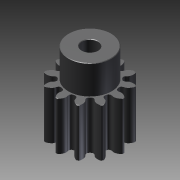
# Autodesk Inventor part: GEAHBB3.0-12-30-B-10_b
Saved by Autodesk Inventor 2011 SP1 (Build 150282100, 282)
## iProperties
Created: 2016-11-09
Part Number: GEAHBB3.0-12-30-B-10_b
Catalog Web Link: www.cadenas.de
Description: GEAHB, GEAHBB, GEAHS, GEAB, GEABB, GEABG, GEAKB, GEAKBB, GEAKBG_3.0_body-Spur Gears - Pressure Angle 20 degree Module 3.0
Vendor: MISUMI
Document SubType Name: Modeling
Designer: psAdmin
Manufacturer: MISUMI
Mass: 35.4987 g
Surface Area: 113.85 cm^2
Volume: 35.4987 cm^3
Density: 1 g/cm^3
Category: PARTsolutions
Company: MISUMI
Title: GEAHBB3.0-12-30-B-10
Author: Cadenas PARTsolutions
Comments: Spur Gears - Pressure Angle 20 degree Module 3.0
PSOL_IDENT_0: {$CADENAS_DATA\23d-libs\misumi\metric\54_spur_gears\geahb30\geahb30.prj},413 {VTYP=3D},{NB=GEAHBB3.0
PSOL_IDENT_1: -12-30-B-10_b},{LINA=GEAHBB3.0-12-30-B-10},{NN=GEAHB, GEAHBB, GEAHS, GEAB, GEABB, GEABG, GEAKB, GEAK
PSOL_IDENT_2: BB, GEAKBG_3.0_body},{DATE=13.09.2016 11:21:23},{GEOMDATE=13.09.2016 06:20:28},{VERSION=},{LINEID=10
PSOL_IDENT_3: },{LINESUBID=-1},{WBVAR=SHS,MAT,ST,NT,TS,PS,ALT1,ALT2,TPC,ALT11,ALT10,BS,ALT4,Z,J,ALT5,Q,R,S,T,ALT9,
PSOL_IDENT_4: SRG,ALT6,LFC,LTC,MALT6,ALT7,KFC,KTC,K,ALT3,DIRALT3,QFC,QTC,MALT3,ALT8,DIRALT8,ZFC,ZTC,U}  {NB=GEAHBB
PSOL_IDENT_5: 3.0-12-30-B-10_b},{LINA=GEAHBB3.0-12-30-B-10},{KT=DUMMY},{PN=GEAHBB3.0-12-30-B-10},{TYPE=GEAHBB},{SH
PSOL_IDENT_6: S=RH},{SHSALG= 'RH','Round Hole','KGH','Key Groove Hole','KGHT','Key Groove Hole+Tap' },{SHALG=1},{S
PSOL_IDENT_7: HSPN=RH},{GEAK=2},{MAT=S45C},{MATALG= 'S45C', 'S45C Equivalent', 'SUS304', 'SUS304' },{ST=BO},{STALG=
PSOL_IDENT_8: '','-','BO','Black Oxide','ENP','Electroless Nickel Plating'},{AC=-},{MOD=3.0},{NT=12},{NTA=[12,14,
PSOL_IDENT_9: 15,16,17,18,19,20,21,22,23,24,25,26,27,28,29,30,32,34,35,36,38,40,42,44,45,46,48,50,52,54,55,56,58,6
PSOL_IDENT_10: 0,62,64,65,68,70]},{B=30},{TS=B},{TSALG='A','A','B','B'},{TSPN=-B},{PS=10},{PSA='8','8','9','9','10'
PSOL_IDENT_11: ,'10','11','11','12','12','13','13','14','14','15','15','16','16','17','17'},{PSA1='8','8','9','9','
PSOL_IDENT_12: 10','10','11','11','12','12','13','13','14','14','15','15','16','16','17','17'},{PSA2='8N','8N','10N'
PSOL_IDENT_13: ,'10N','10K','10K','11N','11N','12N','12N'},{P=10.000},{P2=10},{DD=36.0},{D=42.0},{G=28.5},{H=27},{L=
PSOL_IDENT_14: 48},{LL1=18},{LL2=9},{M=-},{M2=6},{BB=0},{TT=0},{ALT1=},{ALT1ALG= '','N/A' },{ALT1PN=},{ALT2=},{ALT2
PSOL_IDENT_15: ALG= '','N/A' },{TPC=N/A},{TPCALG= 'N/A' },{ALT2PN=},{KC=0},{ALT11=},{ALT11ALG= '','N/A' },{ALT11PN=
PSOL_IDENT_16: },{DEG=0},{ALT10=},{ALT10ALG= '','w/o BS (Boss Cut)','BS','with BS (Boss Cut)' },{BS=0.0},{BSALG=0},
PSOL_IDENT_17: {BSMIN=3},{BSMAX=18},{ALT10PN=},{LL13D=18.000},{LL23D=39.000},{LBS=48.000},{ALT4=},{ALT4ALG='','w/o
PSOL_IDENT_18: Stepped Hole','DHL','with DHL (Stepped Hole)','DHR','with DHR (Stepped Hole)'},{ALT4PN=},{ALT41=1},{
PSOL_IDENT_19: ALT42=1},{Z=0},{ZALG=0},{ZMINL=12},{ZMAXL=24},{ZMINR=12},{ZMAXR=23},{ZPN=},{J=0.0},{JALG=0},{JMIN=2}
PSOL_IDENT_20: ,{JMAX=0},{JPN=},{ALT5=},{ALT5ALG= '','w/o WDH (Both Ends Stepped Hole)','WDH','with WDH (Both Ends
PSOL_IDENT_21: Stepped Hole)' },{ALT5PN=},{Q=0},{QALG=0},{QMIN=12},{QMAX=23},{QPN=},{R=0},{RALG=0},{RMIN=12},{RMAX=
PSOL_IDENT_22: 23},{RPN=},{S=0},{SALG=0},{SMIN=3},{SMAX=42},{SPN=},{T=0},{TALG=0},{TMIN=3},{TMAX=0},{TPN=},{ALT9=},
PSOL_IDENT_23: {ALT9ALG= '','Not applicable' },{SRG=0.0},{SRGALG=0},{SRGMIN=3.500},{SRGMINALG=3.500},{SRGMAX=0.000}
PSOL_IDENT_24: ,{SRGMAXALG=0.000},{DD2=0.0},{MM=0.00},{NN=0.00},{DD2ALG=0.000},{MMALG=0.000},{NNALG=0.000},{ALT9PN=
PSOL_IDENT_25: },{ALT6=},{ALT6ALG= '','Not applicable' },{LFC=0},{LFCALG=0},{LTC=0},{LTCALG=0},{LPCDMIN=18},{LPCDMA
PSOL_IDENT_26: X=21},{MALT6=N/A},{MALT6ALG= 'N/A' },{C=0.0},{ALT6PN=},{ALT7=},{ALT7ALG= '','w/o Side Through Hole','
PSOL_IDENT_27: KFC','with KFC (Side Through Hole)','KTC','with KTC (Side Through Hole)' },{ALT7PN=},{KPCDMIN1=17},{
PSOL_IDENT_28: KPCDMAX1=20},{KPCDMIN2=34},{KPCDMAX2=21},{KFC=0},{KFCALG=[0]},{KTC=0},{KTCALG=[0]},{K=0.0},{KALG=[0]
PSOL_IDENT_29: },{KALT7L=30},{KPCD=0},{TIF=2},{SCREW=0.000},{SCREWL=0},{PLANE=13.5},{PLANE1=13.5},{ALT3=},{ALT3ALG=
PSOL_IDENT_30: '','w/o Side Tapped Hole','QFC','with QFC (Side Tapped Hole)','QTC','with QTC (Side Tapped Hole)' }
PSOL_IDENT_31: ,{ALT3PN=},{DIRALT3=},{DIRALT3ALG= '','N/A' },{QFC=0},{QFCALG=[0]},{QTC=0},{QTCALG=[0]},{QPCDMIN1=17
PSOL_IDENT_32: },{QPCDMAX1=20},{QPCDMIN2=34},{QPCDMAX2=21},{CIFMALT3=3},{QPCD=0},{MALT3=N/A},{MALT3ALG= 'N/A' },{MA
PSOL_IDENT_33: LT3L=0},{PITCH=0},{MS1=3},{ALT8=},{ALT8ALG= '','Not applicable' },{ALT8PN=},{DIRALT8=},{DIRALT8ALG= ''
PSOL_IDENT_34: ,'N/A' },{ZFC=0},{ZFCALG=[0]},{ZTC=0},{ZTCALG=[0]},{ZPCDMIN1=20},{ZPCDMIN2=38},{ZPCDMAX1=16},{ZPCDMA
PSOL_IDENT_35: X2=18},{ZPCD=0},{U=0},{UMAX=0},{UALG=[0]},{UMAX1=0},{UMAX2=6},{UMIN=3},{U1=0.0},{U2=0.0},{F=0.0},{PC
PSOL_IDENT_36: D=0},{PZQRDD2=10},{SHN=0},{SHDEG1=0},{SHDEG2=0},{ALT3LBS=47.5},{ML=0},{MOD3D=3},{D1=7.5},{D2=15},{D3=
PSOL_IDENT_37: 20},{D4=0.3},{D5=6},{D6=3.692308},{D7=2.55},{D8=1.5},{D9=2.406515},{S1=15},{S2=0.5}
NN: 0.00
NT: 12
NB: GEAHBB3.0-12-30-B-10_b
NBSYN: $PN._b
LINA: GEAHBB3.0-12-30-B-10
PN: GEAHBB3.0-12-30-B-10
SHS: Round Hole
MAT: S45C Equivalent
ST: Black Oxide
MOD: 3.0
B: 30
TS: B
PS: 10
DD: 36.0
D: 42.0
G: 28.5
H: 27
L: 48
LL1: 18
LL2: 9
M: -
ALT1: N/A
ALT2: N/A
TPC: N/A
ALT11: N/A
ALT10: w/o BS (Boss Cut)
BS: 0.0
ALT4: w/o Stepped Hole
Z: 0
J: 0.0
ALT5: w/o WDH (Both Ends Stepped Hole)
Q: 0
R: 0
S: 0
T: 0
ALT9: Not applicable
SRG: 0.0
DD2: 0.0
MM: 0.00
ALT6: Not applicable
LFC: 0
LTC: 0
MALT6: N/A
C: 0.0
ALT7: w/o Side Through Hole
KFC: 0
KTC: 0
K: 0.0
ALT3: w/o Side Tapped Hole
DIRALT3: N/A
QFC: 0
QTC: 0
MALT3: N/A
ALT8: Not applicable
DIRALT8: N/A
ZFC: 0
ZTC: 0
U: 0
U1: 0.0
U2: 0.0
F: 0.0
SUPPLIER: MISUMI
ARTICLENO: GEAHBB3.0-12-30-B-10_b
BOMINFO: GEAHBB3.0-12-30-B-10
CREATOR: CADENAS GmbH
Autodesk Inventor part; units mm, degrees
sketch "Sketch_2" plane through (0, 0, 0) normal (1, 0, 0) x (0, 1, 0)
  line L0 (0, -500) -> (0, 500)
  line L1 (0, 48) -> (13.2, 48)
  line L2 (13.2, 48) -> (13.5, 47.7)
  line L3 (13.5, 47.7) -> (13.5, 30)
  line L4 (13.5, 30) -> (20.5, 30)
  line L5 (20.5, 30) -> (26, 28.5263)
  line L6 (26, 28.5263) -> (26, 1.4737)
  line L7 (26, 1.4737) -> (20.5, 0)
  line L8 (20.5, 0) -> (0, 0)
  line L9 (0, 0) -> (0, 48)
  constraints: 20 end point
revolve "Revolution1" add sketch "Sketch_2" angle 360 about axis through (0, 0, -500) along (0, 0, -1)
sketch "Sketch_3" plane through (0, 0, 0) normal (0, 0, 1) x (1, 0, 0)
  circle A0 centre (0, 0) radius 84
  arc A1 (-20.9961, 0.4062) -> (-20.9961, -0.4062) centre (0, 0) ccw
  arc A2 (-20.9961, -0.4062) -> (-20.9145, -0.6061) centre (-20.6961, -0.4004) ccw
  arc A3 (-20.9145, -0.6061) -> (-17.846, -2.3495) centre (-16.5474, 3.5083) ccw
  arc A4 (-17.846, -2.3495) -> (-16.611, -2.2981) centre (-17.3251, 0) ccw
  arc A5 (-15.1899, -2.1473) -> (-16.611, -2.2981) centre (-15.5182, -5.825) ccw
  arc A6 (-13.8639, -3.2946) -> (-15.1899, -2.1473) centre (-15.3233, -3.6414) ccw
  arc A7 (-13.8639, -3.2946) -> (-13.6538, -4.0788) centre (0, 0) ccw
  arc A8 (-14.2285, -5.7353) -> (-13.6538, -4.0788) centre (-15.091, -4.5081) ccw
  arc A9 (-15.5346, -6.3153) -> (-14.2285, -5.7353) centre (-16.3516, -2.7145) ccw
  arc A10 (-15.5346, -6.3153) -> (-16.6298, -6.8883) centre (-15.004, -8.6626) ccw
  arc A11 (-16.6298, -6.8883) -> (-18.4155, -9.9323) centre (-12.5763, -11.312) ccw
  arc A12 (-18.4155, -9.9323) -> (-18.3862, -10.1463) centre (-18.1236, -10.0013) ccw
  arc A13 (-18.3862, -10.1463) -> (-17.98, -10.8498) centre (0, 0) ccw
  arc A14 (-17.98, -10.8498) -> (-17.8094, -10.9821) centre (-17.7232, -10.6948) ccw
  arc A15 (-17.8094, -10.9821) -> (-14.2804, -10.9577) centre (-16.0846, -5.2354) ccw
  arc A16 (-14.2804, -10.9577) -> (-13.2365, -10.2957) centre (-15.004, -8.6626) ccw
  arc A17 (-12.0812, -9.4546) -> (-13.2365, -10.2957) centre (-10.5266, -12.8037) ccw
  arc A18 (-10.3592, -9.7851) -> (-12.0812, -9.4546) centre (-11.4497, -10.8152) ccw
  arc A19 (-10.3592, -9.7851) -> (-9.7851, -10.3592) centre (0, 0) ccw
  arc A20 (-9.4546, -12.0812) -> (-9.7851, -10.3592) centre (-10.8152, -11.4497) ccw
  arc A21 (-10.2957, -13.2365) -> (-9.4546, -12.0812) centre (-12.8037, -10.5266) ccw
  arc A22 (-10.2957, -13.2365) -> (-10.9577, -14.2804) centre (-8.6626, -15.004) ccw
  arc A23 (-10.9577, -14.2804) -> (-10.9821, -17.8094) centre (-5.2354, -16.0846) ccw
  arc A24 (-10.9821, -17.8094) -> (-10.8498, -17.98) centre (-10.6948, -17.7232) ccw
  arc A25 (-10.8498, -17.98) -> (-10.1463, -18.3862) centre (0, 0) ccw
  arc A26 (-10.1463, -18.3862) -> (-9.9323, -18.4155) centre (-10.0013, -18.1236) ccw
  arc A27 (-9.9323, -18.4155) -> (-6.8883, -16.6298) centre (-11.312, -12.5763) ccw
  arc A28 (-6.8883, -16.6298) -> (-6.3153, -15.5346) centre (-8.6626, -15.004) ccw
  arc A29 (-5.7353, -14.2285) -> (-6.3153, -15.5346) centre (-2.7145, -16.3516) ccw
  arc A30 (-4.0788, -13.6538) -> (-5.7353, -14.2285) centre (-4.5081, -15.091) ccw
  arc A31 (-4.0788, -13.6538) -> (-3.2946, -13.8639) centre (0, 0) ccw
  arc A32 (-2.1473, -15.1899) -> (-3.2946, -13.8639) centre (-3.6414, -15.3233) ccw
  arc A33 (-2.2981, -16.611) -> (-2.1473, -15.1899) centre (-5.825, -15.5182) ccw
  arc A34 (-2.2981, -16.611) -> (-2.3495, -17.846) centre (0, -17.3251) ccw
  arc A35 (-2.3495, -17.846) -> (-0.6061, -20.9145) centre (3.5083, -16.5474) ccw
  arc A36 (-0.6061, -20.9145) -> (-0.4062, -20.9961) centre (-0.4004, -20.6961) ccw
  arc A37 (-0.4062, -20.9961) -> (0.4062, -20.9961) centre (0, 0) ccw
  arc A38 (0.4062, -20.9961) -> (0.6061, -20.9145) centre (0.4004, -20.6961) ccw
  arc A39 (0.6061, -20.9145) -> (2.3495, -17.846) centre (-3.5083, -16.5474) ccw
  arc A40 (2.3495, -17.846) -> (2.2981, -16.611) centre (0, -17.3251) ccw
  arc A41 (2.1473, -15.1899) -> (2.2981, -16.611) centre (5.825, -15.5182) ccw
  arc A42 (3.2946, -13.8639) -> (2.1473, -15.1899) centre (3.6414, -15.3233) ccw
  arc A43 (3.2946, -13.8639) -> (4.0788, -13.6538) centre (0, 0) ccw
  arc A44 (5.7353, -14.2285) -> (4.0788, -13.6538) centre (4.5081, -15.091) ccw
  arc A45 (6.3153, -15.5346) -> (5.7353, -14.2285) centre (2.7145, -16.3516) ccw
  arc A46 (6.3153, -15.5346) -> (6.8883, -16.6298) centre (8.6626, -15.004) ccw
  arc A47 (6.8883, -16.6298) -> (9.9323, -18.4155) centre (11.312, -12.5763) ccw
  arc A48 (9.9323, -18.4155) -> (10.1463, -18.3862) centre (10.0013, -18.1236) ccw
  arc A49 (10.1463, -18.3862) -> (10.8498, -17.98) centre (0, 0) ccw
  arc A50 (10.8498, -17.98) -> (10.9821, -17.8094) centre (10.6948, -17.7232) ccw
  arc A51 (10.9821, -17.8094) -> (10.9577, -14.2804) centre (5.2354, -16.0846) ccw
  arc A52 (10.9577, -14.2804) -> (10.2957, -13.2365) centre (8.6626, -15.004) ccw
  arc A53 (9.4546, -12.0812) -> (10.2957, -13.2365) centre (12.8037, -10.5266) ccw
  arc A54 (9.7851, -10.3592) -> (9.4546, -12.0812) centre (10.8152, -11.4497) ccw
  arc A55 (9.7851, -10.3592) -> (10.3592, -9.7851) centre (0, 0) ccw
  arc A56 (12.0812, -9.4546) -> (10.3592, -9.7851) centre (11.4497, -10.8152) ccw
  arc A57 (13.2365, -10.2957) -> (12.0812, -9.4546) centre (10.5266, -12.8037) ccw
  arc A58 (13.2365, -10.2957) -> (14.2804, -10.9577) centre (15.004, -8.6626) ccw
  arc A59 (14.2804, -10.9577) -> (17.8094, -10.9821) centre (16.0846, -5.2354) ccw
  arc A60 (17.8094, -10.9821) -> (17.98, -10.8498) centre (17.7232, -10.6948) ccw
  arc A61 (17.98, -10.8498) -> (18.3862, -10.1463) centre (0, 0) ccw
  arc A62 (18.3862, -10.1463) -> (18.4155, -9.9323) centre (18.1236, -10.0013) ccw
  arc A63 (18.4155, -9.9323) -> (16.6298, -6.8883) centre (12.5763, -11.312) ccw
  arc A64 (16.6298, -6.8883) -> (15.5346, -6.3153) centre (15.004, -8.6626) ccw
  arc A65 (14.2285, -5.7353) -> (15.5346, -6.3153) centre (16.3516, -2.7145) ccw
  arc A66 (13.6538, -4.0788) -> (14.2285, -5.7353) centre (15.091, -4.5081) ccw
  arc A67 (13.6538, -4.0788) -> (13.8639, -3.2946) centre (0, 0) ccw
  arc A68 (15.1899, -2.1473) -> (13.8639, -3.2946) centre (15.3233, -3.6414) ccw
  arc A69 (16.611, -2.2981) -> (15.1899, -2.1473) centre (15.5182, -5.825) ccw
  arc A70 (16.611, -2.2981) -> (17.846, -2.3495) centre (17.3251, 0) ccw
  arc A71 (17.846, -2.3495) -> (20.9145, -0.6061) centre (16.5474, 3.5083) ccw
  arc A72 (20.9145, -0.6061) -> (20.9961, -0.4062) centre (20.6961, -0.4004) ccw
  arc A73 (20.9961, -0.4062) -> (20.9961, 0.4062) centre (0, 0) ccw
  arc A74 (20.9961, 0.4062) -> (20.9145, 0.6061) centre (20.6961, 0.4004) ccw
  arc A75 (20.9145, 0.6061) -> (17.846, 2.3495) centre (16.5474, -3.5083) ccw
  arc A76 (17.846, 2.3495) -> (16.611, 2.2981) centre (17.3251, 0) ccw
  arc A77 (15.1899, 2.1473) -> (16.611, 2.2981) centre (15.5182, 5.825) ccw
  arc A78 (13.8639, 3.2946) -> (15.1899, 2.1473) centre (15.3233, 3.6414) ccw
  arc A79 (13.8639, 3.2946) -> (13.6538, 4.0788) centre (0, 0) ccw
  arc A80 (14.2285, 5.7353) -> (13.6538, 4.0788) centre (15.091, 4.5081) ccw
  arc A81 (15.5346, 6.3153) -> (14.2285, 5.7353) centre (16.3516, 2.7145) ccw
  arc A82 (15.5346, 6.3153) -> (16.6298, 6.8883) centre (15.004, 8.6626) ccw
  arc A83 (16.6298, 6.8883) -> (18.4155, 9.9323) centre (12.5763, 11.312) ccw
  arc A84 (18.4155, 9.9323) -> (18.3862, 10.1463) centre (18.1236, 10.0013) ccw
  arc A85 (18.3862, 10.1463) -> (17.98, 10.8498) centre (0, 0) ccw
  arc A86 (17.98, 10.8498) -> (17.8094, 10.9821) centre (17.7232, 10.6948) ccw
  arc A87 (17.8094, 10.9821) -> (14.2804, 10.9577) centre (16.0846, 5.2354) ccw
  arc A88 (14.2804, 10.9577) -> (13.2365, 10.2957) centre (15.004, 8.6626) ccw
  arc A89 (12.0812, 9.4546) -> (13.2365, 10.2957) centre (10.5266, 12.8037) ccw
  arc A90 (10.3592, 9.7851) -> (12.0812, 9.4546) centre (11.4497, 10.8152) ccw
  arc A91 (10.3592, 9.7851) -> (9.7851, 10.3592) centre (0, 0) ccw
  arc A92 (9.4546, 12.0812) -> (9.7851, 10.3592) centre (10.8152, 11.4497) ccw
  arc A93 (10.2957, 13.2365) -> (9.4546, 12.0812) centre (12.8037, 10.5266) ccw
  arc A94 (10.2957, 13.2365) -> (10.9577, 14.2804) centre (8.6626, 15.004) ccw
  arc A95 (10.9577, 14.2804) -> (10.9821, 17.8094) centre (5.2354, 16.0846) ccw
  arc A96 (10.9821, 17.8094) -> (10.8498, 17.98) centre (10.6948, 17.7232) ccw
  arc A97 (10.8498, 17.98) -> (10.1463, 18.3862) centre (0, 0) ccw
  arc A98 (10.1463, 18.3862) -> (9.9323, 18.4155) centre (10.0013, 18.1236) ccw
  arc A99 (9.9323, 18.4155) -> (6.8883, 16.6298) centre (11.312, 12.5763) ccw
  arc A100 (6.8883, 16.6298) -> (6.3153, 15.5346) centre (8.6626, 15.004) ccw
  arc A101 (5.7353, 14.2285) -> (6.3153, 15.5346) centre (2.7145, 16.3516) ccw
  arc A102 (4.0788, 13.6538) -> (5.7353, 14.2285) centre (4.5081, 15.091) ccw
  arc A103 (4.0788, 13.6538) -> (3.2946, 13.8639) centre (0, 0) ccw
  arc A104 (2.1473, 15.1899) -> (3.2946, 13.8639) centre (3.6414, 15.3233) ccw
  arc A105 (2.2981, 16.611) -> (2.1473, 15.1899) centre (5.825, 15.5182) ccw
  arc A106 (2.2981, 16.611) -> (2.3495, 17.846) centre (0, 17.3251) ccw
  arc A107 (2.3495, 17.846) -> (0.6061, 20.9145) centre (-3.5083, 16.5474) ccw
  arc A108 (0.6061, 20.9145) -> (0.4062, 20.9961) centre (0.4004, 20.6961) ccw
  arc A109 (0.4062, 20.9961) -> (-0.4062, 20.9961) centre (0, 0) ccw
  arc A110 (-0.4062, 20.9961) -> (-0.6061, 20.9145) centre (-0.4004, 20.6961) ccw
  arc A111 (-0.6061, 20.9145) -> (-2.3495, 17.846) centre (3.5083, 16.5474) ccw
  arc A112 (-2.3495, 17.846) -> (-2.2981, 16.611) centre (0, 17.3251) ccw
  arc A113 (-2.1473, 15.1899) -> (-2.2981, 16.611) centre (-5.825, 15.5182) ccw
  arc A114 (-3.2946, 13.8639) -> (-2.1473, 15.1899) centre (-3.6414, 15.3233) ccw
  arc A115 (-3.2946, 13.8639) -> (-4.0788, 13.6538) centre (0, 0) ccw
  arc A116 (-5.7353, 14.2285) -> (-4.0788, 13.6538) centre (-4.5081, 15.091) ccw
  arc A117 (-6.3153, 15.5346) -> (-5.7353, 14.2285) centre (-2.7145, 16.3516) ccw
  arc A118 (-6.3153, 15.5346) -> (-6.8883, 16.6298) centre (-8.6626, 15.004) ccw
  arc A119 (-6.8883, 16.6298) -> (-9.9323, 18.4155) centre (-11.312, 12.5763) ccw
  arc A120 (-9.9323, 18.4155) -> (-10.1463, 18.3862) centre (-10.0013, 18.1236) ccw
  arc A121 (-10.1463, 18.3862) -> (-10.8498, 17.98) centre (0, 0) ccw
  arc A122 (-10.8498, 17.98) -> (-10.9821, 17.8094) centre (-10.6948, 17.7232) ccw
  arc A123 (-10.9821, 17.8094) -> (-10.9577, 14.2804) centre (-5.2354, 16.0846) ccw
  arc A124 (-10.9577, 14.2804) -> (-10.2957, 13.2365) centre (-8.6626, 15.004) ccw
  arc A125 (-9.4546, 12.0812) -> (-10.2957, 13.2365) centre (-12.8037, 10.5266) ccw
  arc A126 (-9.7851, 10.3592) -> (-9.4546, 12.0812) centre (-10.8152, 11.4497) ccw
  arc A127 (-9.7851, 10.3592) -> (-10.3592, 9.7851) centre (0, 0) ccw
  arc A128 (-12.0812, 9.4546) -> (-10.3592, 9.7851) centre (-11.4497, 10.8152) ccw
  arc A129 (-13.2365, 10.2957) -> (-12.0812, 9.4546) centre (-10.5266, 12.8037) ccw
  arc A130 (-13.2365, 10.2957) -> (-14.2804, 10.9577) centre (-15.004, 8.6626) ccw
  arc A131 (-14.2804, 10.9577) -> (-17.8094, 10.9821) centre (-16.0846, 5.2354) ccw
  arc A132 (-17.8094, 10.9821) -> (-17.98, 10.8498) centre (-17.7232, 10.6948) ccw
  arc A133 (-17.98, 10.8498) -> (-18.3862, 10.1463) centre (0, 0) ccw
  arc A134 (-18.3862, 10.1463) -> (-18.4155, 9.9323) centre (-18.1236, 10.0013) ccw
  arc A135 (-18.4155, 9.9323) -> (-16.6298, 6.8883) centre (-12.5763, 11.312) ccw
  arc A136 (-16.6298, 6.8883) -> (-15.5346, 6.3153) centre (-15.004, 8.6626) ccw
  arc A137 (-14.2285, 5.7353) -> (-15.5346, 6.3153) centre (-16.3516, 2.7145) ccw
  arc A138 (-13.6538, 4.0788) -> (-14.2285, 5.7353) centre (-15.091, 4.5081) ccw
  arc A139 (-13.6538, 4.0788) -> (-13.8639, 3.2946) centre (0, 0) ccw
  arc A140 (-15.1899, 2.1473) -> (-13.8639, 3.2946) centre (-15.3233, 3.6414) ccw
  arc A141 (-16.611, 2.2981) -> (-15.1899, 2.1473) centre (-15.5182, 5.825) ccw
  arc A142 (-16.611, 2.2981) -> (-17.846, 2.3495) centre (-17.3251, 0) ccw
  arc A143 (-17.846, 2.3495) -> (-20.9145, 0.6061) centre (-16.5474, -3.5083) ccw
  arc A144 (-20.9145, 0.6061) -> (-20.9961, 0.4062) centre (-20.6961, 0.4004) ccw
  constraints: 288 point on circle, 145 centre point
extrude "Extrusion1" cut sketch "Sketch_3" along normal blind 30
sketch "Sketch3" plane through (-12.5763, 11.312, 0) normal (0, 0, -1) x (-0.8357, -0.5492, 0)
  point P0 (-4.2979, -16.3601)
hole "Hole1" at (0, 0, 0) direction (0, 0, 1) diameter 10 depth 48
sketch "_____5" plane through (0, 0, 0) normal (1, 0, 0) x (0, 0, -1)
  line L0 (500, 0) -> (-500, 0)
  line L1 (-0.3, 5) -> (0, 5)
  line L2 (0, 5) -> (0, 5.3)
  line L3 (0, 5.3) -> (-0.3, 5)
  constraints: 8 end point
revolve "Revolution2" cut sketch "_____5" angle 360 about axis through (0, 0, -500) along (0, 0, -1)
sketch "_____7" plane through (0, 0, 0) normal (1, 0, 0) x (0, 0, -1)
  line L0 (500, 0) -> (-500, 0)
  line L1 (-48, 5) -> (-47.7, 5)
  line L2 (-47.7, 5) -> (-48, 5.3)
  line L3 (-48, 5.3) -> (-48, 5)
  constraints: 8 end point
revolve "Revolution3" cut sketch "_____7" angle 360 about axis through (0, 0, -500) along (0, 0, -1)
ref_plane "b_XY" through (0, 0, 0) normal (0, 0, 1) x (1, 0, 0)
ref_plane "b_YZ" through (0, 0, 0) normal (1, 0, 0) x (0, 1, 0)
ref_plane "b_ZX" through (0, 0, 0) normal (0, 1, 0) x (0, 0, 1)
ref_plane "turn_around_XY" through (0, 0, 0) normal (-1, 0, 0) x (0, 0, -1)
ref_plane "turn_around_YZ" through (0, 0, 0) normal (0, 0, -1) x (0, -1, 0)
ref_plane "turn_around_ZX" through (0, 0, 0) normal (0, -1, 0) x (-1, 0, 0)
body "Solid1"
